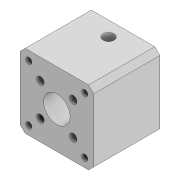
# Autodesk Inventor part: Part1_b
Saved by Autodesk Inventor 2021 (Build 250183000, 183)
## iProperties
Created: 2022-05-23
Part Number: Part1_b
Material: Generic
Document SubType Name: Modeling
Designer: romanp
Density: 1 g/cm^3
Appearance: Default
Author: romanp
Autodesk Inventor part; units mm, degrees
ref_plane "YZ Plane" through (0, 0, 0) normal (1, 0, 0) x (0, 1, 0)
ref_plane "XZ Plane" through (0, 0, 0) normal (0, 1, 0) x (-1, 0, 0)
ref_plane "XY Plane" through (0, 0, 0) normal (0, 0, 1) x (1, 0, 0)
sketch "Sketch11" plane through (0, 0, 0) normal (0, 0, 1) x (1, 0, 0)
  line L0 (-3.4593, 3.4593) -> (0, 0)
  line L1 (-3.4593, 3.4593) -> (-3.4593, 46.5407)
  line L2 (0, 50) -> (-3.4593, 46.5407)
  line L3 (43.0814, 50) -> (0, 50)
  line L4 (46.5407, 46.5407) -> (43.0814, 50)
  line L5 (46.5407, 3.4593) -> (46.5407, 46.5407)
  line L6 (43.0814, 0) -> (46.5407, 3.4593)
  line L7 (43.0814, 0) -> (0, 0)
  constraints: 16 end point
extrude "Extrusion8" add sketch "Sketch11" along normal blind 5
sketch "Sketch16" plane through (0, 0, 0) normal (0, 0, -1) x (-1, 0, 0)
  line L0 (-27.0407, 40) -> (-34.0407, 40)
  line L1 (-36.5407, 37.5) -> (-36.5407, 30.5)
  arc A0 (-34.0407, 40) -> (-36.5407, 37.5) centre (-34.0407, 37.5) ccw
  line L2 (-9.0407, 40) -> (-16.0407, 40)
  arc A1 (-6.5407, 37.5) -> (-9.0407, 40) centre (-9.0407, 37.5) ccw
  line L3 (-6.5407, 30.5) -> (-6.5407, 37.5)
  line L4 (-6.5407, 12.5) -> (-6.5407, 19.5)
  arc A2 (-9.0407, 10) -> (-6.5407, 12.5) centre (-9.0407, 12.5) ccw
  line L5 (-16.0407, 10) -> (-9.0407, 10)
  line L6 (-34.0407, 10) -> (-27.0407, 10)
  arc A3 (-36.5407, 12.5) -> (-34.0407, 10) centre (-34.0407, 12.5) ccw
  line L7 (-36.5407, 19.5) -> (-36.5407, 12.5)
  line L8 (0, 50) -> (3.4593, 46.5407) projected
  line L9 (-43.0814, 0) -> (-46.5407, 3.4593) projected
  line L10 (-46.5407, 46.5407) -> (-43.0814, 50) projected
  line L11 (-43.0814, 0) -> (-43.0814, 50)
  line L12 (3.4593, 3.4593) -> (0, 0) projected
  line L13 (-6.5407, 30.5) -> (-6.5407, 19.5)
  line L14 (-16.0407, 40) -> (-27.0407, 40)
  line L15 (-36.5407, 30.5) -> (-36.5407, 19.5)
  line L16 (-27.0407, 10) -> (-16.0407, 10)
  circle A4 centre (-2.5407, 44) radius 2.5
  circle A5 centre (-40.5407, 6) radius 2.5
  circle A6 centre (-2.5407, 6) radius 2.5
  circle A7 centre (-40.5407, 44) radius 2.5
  line L17 (0, 50) -> (3.4593, 46.5407)
  line L18 (3.4593, 46.5407) -> (3.4593, 3.4593) projected
  line L19 (0, 0) -> (-43.0814, 0) projected
  line L20 (3.4593, 3.4593) -> (0, 0)
  line L21 (0, 0) -> (-43.0814, 0)
  line L22 (-43.0814, 0) -> (-46.5407, 3.4593) projected
  line L23 (-43.0814, 0) -> (-46.5407, 3.4593)
  line L24 (-46.5407, 3.4593) -> (-46.5407, 46.5407) projected
  line L25 (-46.5407, 3.4593) -> (-46.5407, 46.5407)
  line L26 (-46.5407, 46.5407) -> (-43.0814, 50)
  line L27 (0, 50) -> (-43.0814, 50) projected
  line L28 (0, 50) -> (-43.0814, 50)
  dimension "d44" = 5
  dimension "d45" = 5
  dimension "d46" = 5
  dimension "d47" = 5
  constraints: 40 end point, 8 centre point, 8 collinear, 8 point on circle, 2 vertical, 1 perpendicular, 1 point on line
  measures "d44" diameter of A4
  measures "d45" diameter of A5
  measures "d46" diameter of A6
  measures "d47" diameter of A7
extrude "Extrusion11" add sketch "Sketch16" along normal blind 15
sketch "Sketch18" plane through (0, 0, -15) normal (0, 0, -1) x (-1, 0, 0)
  circle A0 centre (-2.5407, 6) radius 2.5 projected
  circle A1 centre (-2.5407, 6) radius 2.5
  circle A2 centre (-40.5407, 6) radius 2.5 projected
  circle A3 centre (-40.5407, 6) radius 2.5
  circle A4 centre (-40.5407, 44) radius 2.5 projected
  circle A5 centre (-40.5407, 44) radius 2.5
  circle A6 centre (-2.5407, 44) radius 2.5 projected
  circle A7 centre (-2.5407, 44) radius 2.5
  point P0 (0, 0)
  constraints: 4 centre point, 4 coincident
extrude "Extrusion12" cut sketch "Sketch18" against normal blind 100
sketch "Sketch19" plane through (0, 0, -15) normal (0, 0, -1) x (-1, 0, 0)
  circle A0 centre (-2.5407, 6) radius 2.5 projected
  circle A1 centre (-2.5407, 6) radius 4.3
  circle A2 centre (-40.5407, 6) radius 2.5 projected
  circle A3 centre (-40.5407, 6) radius 4.3
  circle A4 centre (-2.5407, 44) radius 2.5 projected
  circle A5 centre (-2.5407, 44) radius 4.3
  circle A6 centre (-40.5407, 44) radius 2.5 projected
  circle A7 centre (-40.5407, 44) radius 4.3
  point P0 (0, 0)
  dimension "d54" = 8.6
  dimension "d55" = 8.6
  dimension "d56" = 8.6
  dimension "d57" = 8.6
  constraints: 4 centre point, 4 coincident
  measures "d54" diameter of A1
  measures "d55" diameter of A3
  measures "d56" diameter of A5
  measures "d57" diameter of A7
extrude "Extrusion13" cut sketch "Sketch19" against normal blind 10 contours A0 | A1 | A2 | A3 | A5 | A6 | A7
sketch "Sketch20" plane through (0, 0, -15) normal (0, 0, -1) x (-1, 0, 0)
  line L0 (0, 50) -> (-43.0814, 50) projected
  line L1 (-43.0814, 50) -> (-46.5407, 46.5407) projected
  line L2 (-46.5407, 46.5407) -> (-46.5407, 3.4593) projected
  line L3 (-46.5407, 3.4593) -> (-43.0814, 0) projected
  line L4 (-43.0814, 0) -> (0, 0) projected
  line L5 (0, 0) -> (3.4593, 3.4593) projected
  line L6 (3.4593, 3.4593) -> (3.4593, 46.5407) projected
  line L7 (3.4593, 46.5407) -> (0, 50) projected
  circle A0 centre (-2.5407, 44) radius 4.3 projected
  circle A1 centre (-40.5407, 44) radius 4.3 projected
  circle A2 centre (-40.5407, 6) radius 4.3 projected
  circle A3 centre (-2.5407, 6) radius 4.3 projected
  arc A4 (-9.0407, 10) -> (-6.5407, 12.5) centre (-9.0407, 12.5) ccw projected
  line L8 (-9.0407, 10) -> (-34.0407, 10) projected
  line L9 (-36.5407, 12.5) -> (-36.5407, 37.5) projected
  arc A5 (-36.5407, 12.5) -> (-34.0407, 10) centre (-34.0407, 12.5) ccw projected
  line L10 (-6.5407, 37.5) -> (-6.5407, 12.5) projected
  arc A6 (-6.5407, 37.5) -> (-9.0407, 40) centre (-9.0407, 37.5) ccw projected
  line L11 (-34.0407, 40) -> (-9.0407, 40) projected
  arc A7 (-34.0407, 40) -> (-36.5407, 37.5) centre (-34.0407, 37.5) ccw projected
extrude "Extrusion14" add sketch "Sketch20" along normal blind 25
sketch "Sketch21" plane through (0, 50, 5) normal (0, 1, 0) x (1, 0, 0)
  line L0 (-1.7593, 45) -> (6.8407, 45) projected
  circle A0 centre (21.6907, 35) radius 2
  dimension "d63" = 4
  constraints: 1 centre point
  measures "d63" diameter of A0
extrude "Extrusion15" cut sketch "Sketch21" against normal blind 500
sketch "Sketch22" plane through (0, 50, 5) normal (0, 1, 0) x (1, 0, 0)
  circle A0 centre (21.6907, 35) radius 2 projected
  circle A1 centre (21.6907, 35) radius 3.75
  point P0 (0, 5)
  dimension "d67" = 7.5
  constraints: 1 centre point, 1 coincident
  measures "d67" diameter of A1
extrude "Extrusion16" cut sketch "Sketch22" against normal blind 5 contours A0 | A1
sketch "Sketch23" plane through (0, 0, 5) normal (0, -1, 0) x (1, 0, 0)
  circle A0 centre (21.6907, -35) radius 2 projected
  circle A1 centre (21.6907, -35) radius 3.75
  point P0 (0, -5)
  dimension "d70" = 7.5
  constraints: 1 centre point, 1 coincident
  measures "d70" diameter of A1
extrude "Extrusion17" cut sketch "Sketch23" against normal blind 5
sketch "Sketch25" plane through (2.5407, 44, -5) normal (0, 0, -1) x (-1, 0, 0)
  circle A0 centre (0, 0) radius 2.5 projected
  circle A1 centre (0, -38) radius 2.5 projected
  circle A2 centre (-38, -38) radius 2.5 projected
  circle A3 centre (-38, 0) radius 2.5 projected
  circle A4 centre (0, 0) radius 2
  circle A5 centre (0, -38) radius 2.5 projected
  circle A6 centre (0, -38) radius 2
  circle A7 centre (-38, -38) radius 2
  circle A8 centre (-38, 0) radius 2
  point P0 (2.5407, -44)
  dimension "d75" = 4
  dimension "d76" = 4
  dimension "d77" = 4
  dimension "d78" = 4
  constraints: 4 centre point, 4 coincident
  measures "d75" diameter of A4
  measures "d76" diameter of A6
  measures "d77" diameter of A7
  measures "d78" diameter of A8
extrude "Extrusion18" add sketch "Sketch25" against normal blind 10
sketch "Sketch26" plane through (0, 0, -40) normal (0, 0, -1) x (-1, 0, 0)
  circle A0 centre (-2.5407, 44) radius 4.3 projected
  circle A1 centre (-2.5407, 6) radius 4.3 projected
  circle A2 centre (-40.5407, 6) radius 4.3 projected
  circle A3 centre (-40.5407, 44) radius 4.3 projected
  circle A4 centre (-2.5407, 6) radius 2 projected
  circle A5 centre (-2.5407, 6) radius 3.8
  circle A6 centre (-40.5407, 6) radius 4.3 projected
  circle A7 centre (-40.5407, 6) radius 3.8
  circle A8 centre (-2.5407, 44) radius 2 projected
  circle A9 centre (-2.5407, 44) radius 3.8
  circle A10 centre (-40.5407, 44) radius 2 projected
  circle A11 centre (-40.5407, 44) radius 3.8
  point P0 (0, 0)
  dimension "d81" = 7.6
  dimension "d82" = 7.6
  dimension "d83" = 7.6
  dimension "d84" = 7.6
  constraints: 4 centre point, 4 coincident
  measures "d81" diameter of A5
  measures "d82" diameter of A7
  measures "d83" diameter of A9
  measures "d84" diameter of A11
extrude "Extrusion19" add sketch "Sketch26" against normal blind 35 contours A0 | A1 | A2 | A3
sketch "Sketch27" plane through (0, 0, 5) normal (0, 0, 1) x (1, 0, 0)
  circle A0 centre (2.5407, 44) radius 2 projected
  circle A1 centre (40.5407, 44) radius 2 projected
  circle A2 centre (2.5407, 6) radius 2 projected
  circle A3 centre (40.5407, 6) radius 2 projected
  circle A4 centre (21.5407, 25) radius 9
  point P0 (0, 0)
  dimension "d88" = 18
  constraints: 1 centre point
  measures "d88" diameter of A4
extrude "Extrusion20" cut sketch "Sketch27" against normal blind 35 contours A4
sketch "Sketch32" plane through (0, 0, -40) normal (0, 0, -1) x (-1, 0, 0)
  circle A0 centre (-21.5407, 25) radius 9 projected
  circle A1 centre (-2.5407, 6) radius 2 projected
  circle A2 centre (-40.5407, 44) radius 2 projected
  circle A3 centre (-2.5407, 44) radius 2 projected
  circle A4 centre (-40.5407, 6) radius 2 projected
  circle A5 centre (-10.4038, 13.8631) radius 2.5
  circle A6 centre (-32.6776, 13.8631) radius 2.5
  circle A7 centre (-10.4038, 36.1369) radius 2.5
  circle A8 centre (-32.6776, 36.1369) radius 2.5
  point P0 (0, 0)
  dimension "d93" = 5
  dimension "d94" = 5
  dimension "d95" = 5
  dimension "d96" = 5
  constraints: 4 centre point
  measures "d93" diameter of A5
  measures "d94" diameter of A6
  measures "d95" diameter of A7
  measures "d96" diameter of A8
extrude "Extrusion21" cut sketch "Sketch32" against normal blind 100 contours A5 | A6 | A7 | A8
sketch "Sketch33" plane through (0, 0, 0) normal (0, 0, -1) x (-1, 0, 0)
  circle A0 centre (-10.4038, 13.8631) radius 2.5 projected
  circle A1 centre (-10.4038, 13.8631) radius 4.5
  circle A2 centre (-10.4038, 36.1369) radius 2.5 projected
  circle A3 centre (-10.4038, 36.1369) radius 4.5
  circle A4 centre (-32.6776, 36.1369) radius 2.5 projected
  circle A5 centre (-32.6776, 36.1369) radius 4.5
  circle A6 centre (-32.6776, 13.8631) radius 2.5 projected
  circle A7 centre (-32.6776, 13.8631) radius 4.5
  point P0 (0, 0)
  dimension "d99" = 9
  dimension "d100" = 9
  dimension "d101" = 9
  dimension "d102" = 9
  constraints: 4 centre point, 4 coincident
  measures "d99" diameter of A1
  measures "d100" diameter of A3
  measures "d101" diameter of A5
  measures "d102" diameter of A7
extrude "Extrusion22" cut sketch "Sketch33" along normal blind 100 and the other way blind 5
sketch "Sketch34" plane through (0, 0, 5) normal (0, 0, 1) x (1, 0, 0)
  circle A0 centre (10.4038, 36.1369) radius 4.5 projected
  circle A1 centre (10.4038, 36.1369) radius 2.5
  arc A2 (30.3697, 40) -> (36.5407, 33.829) centre (32.6776, 36.1369) ccw projected
  circle A3 centre (32.6776, 36.1369) radius 2.5
  circle A4 centre (10.4038, 13.8631) radius 4.5 projected
  circle A5 centre (10.4038, 13.8631) radius 2.5
  circle A6 centre (32.6776, 13.8631) radius 4.5 projected
  circle A7 centre (32.6776, 13.8631) radius 2.5
  circle A8 centre (32.6776, 36.1369) radius 4.5 projected
  point P0 (0, 0)
  dimension "d107" = 5
  dimension "d108" = 5
  dimension "d109" = 5
  dimension "d110" = 5
  constraints: 4 centre point, 4 coincident
  measures "d107" diameter of A1
  measures "d108" diameter of A3
  measures "d109" diameter of A5
  measures "d110" diameter of A7
extrude "Extrusion23" add sketch "Sketch34" against normal blind 5
sketch "Sketch35" plane through (0, 0, 0) normal (0, 0, -1) x (-1, 0, 0)
  circle A0 centre (-32.6776, 13.8631) radius 2.5 projected
  circle A1 centre (-32.6776, 36.1369) radius 2.5 projected
  circle A2 centre (-10.4038, 13.8631) radius 2.5 projected
  circle A3 centre (-10.4038, 36.1369) radius 2.5 projected
  line L0 (-30.3697, 10) -> (-12.7117, 10) projected
  arc A4 (-12.7117, 10) -> (-6.5407, 16.171) centre (-10.4038, 13.8631) ccw projected
  line L1 (-6.5407, 16.171) -> (-6.5407, 33.829) projected
  arc A5 (-6.5407, 33.829) -> (-12.7117, 40) centre (-10.4038, 36.1369) ccw projected
  line L2 (-12.7117, 40) -> (-30.3697, 40) projected
  arc A6 (-30.3697, 40) -> (-36.5407, 33.829) centre (-32.6776, 36.1369) ccw projected
  line L3 (-36.5407, 33.829) -> (-36.5407, 16.171) projected
  arc A7 (-36.5407, 16.171) -> (-30.3697, 10) centre (-32.6776, 13.8631) ccw projected
  circle A8 centre (-21.5407, 25) radius 9 projected
  circle A9 centre (-32.6776, 36.1369) radius 4.5
  circle A10 centre (-10.4038, 36.1369) radius 2.5 projected
  circle A11 centre (-10.4038, 36.1369) radius 4.5
  circle A12 centre (-32.6776, 13.8631) radius 4.5
  circle A13 centre (-10.4038, 13.8631) radius 2.5 projected
  arc A14 (-12.7117, 10) -> (-6.5407, 16.171) centre (-10.4038, 13.8631) ccw projected
  circle A15 centre (-10.4038, 13.8631) radius 4.5
  point P0 (0, 0)
  point P1 (-12.7117, 40)
  constraints: 4 coincident, 2 centre point, 6 other
extrude "Extrusion24" add sketch "Sketch35" along normal blind 10 contours A12 L3 A9 L2 A11 L1 A15 L0
sketch "Sketch37" plane through (40.5407, 44, -5) normal (0, 0, -1) x (-1, 0, 0)
  circle A0 centre (0, 0) radius 3.8 projected
  circle A1 centre (0, 0) radius 2 projected
  circle A2 centre (38, 0) radius 3.8 projected
  circle A3 centre (38, 0) radius 2 projected
  circle A4 centre (38, -38) radius 3.8 projected
  circle A5 centre (38, -38) radius 2 projected
  circle A6 centre (0, -38) radius 3.8 projected
  circle A7 centre (0, -38) radius 2 projected
  point P0 (40.5407, -44)
extrude "Extrusion25" add sketch "Sketch37" along normal blind 2
sketch "Sketch38" plane through (0, 0, -40) normal (0, 0, -1) x (-1, 0, 0)
  line L0 (-6.5407, 33.829) -> (-6.5407, 16.171) projected
  arc A0 (-12.7117, 40) -> (-6.5407, 33.829) centre (-10.4038, 36.1369) ccw projected
  line L1 (-30.3697, 40) -> (-12.7117, 40) projected
  arc A1 (-36.5407, 33.829) -> (-30.3697, 40) centre (-32.6776, 36.1369) ccw projected
  line L2 (-36.5407, 16.171) -> (-36.5407, 33.829) projected
  arc A2 (-30.3697, 10) -> (-36.5407, 16.171) centre (-32.6776, 13.8631) ccw projected
  line L3 (-12.7117, 10) -> (-30.3697, 10) projected
  arc A3 (-6.5407, 16.171) -> (-12.7117, 10) centre (-10.4038, 13.8631) ccw projected
  circle A4 centre (-21.5407, 25) radius 9 projected
  arc A5 (-30.3697, 40) -> (-36.5407, 33.829) centre (-32.6776, 36.1369) ccw projected
  arc A6 (-36.5407, 16.171) -> (-30.3697, 10) centre (-32.6776, 13.8631) ccw projected
  arc A7 (-6.5407, 33.829) -> (-12.7117, 40) centre (-10.4038, 36.1369) ccw projected
  line L4 (-36.5407, 16.171) -> (-36.5407, 33.829) projected
  arc A8 (-12.7117, 10) -> (-6.5407, 16.171) centre (-10.4038, 13.8631) ccw projected
  line L5 (-21.5407, 25) -> (-36.7907, 25)
  line L6 (-36.7907, 25) -> (-36.7907, 9.75)
  line L7 (-21.5407, 25) -> (-6.2907, 25)
  line L8 (-6.2907, 25) -> (-6.2907, 40.25)
  line L9 (-36.7907, 9.75) -> (-6.2907, 9.75)
  line L10 (-6.2907, 9.75) -> (-6.2907, 40.25)
  line L11 (-6.2907, 40.25) -> (-36.7907, 40.25)
  line L12 (-36.7907, 40.25) -> (-36.7907, 9.75)
  point P0 (0, 0)
  point P1 (-6.2907, 15.6886)
  point P2 (-6.2907, 34.3114)
  point P3 (-30.8521, 9.75)
  point P4 (-12.2293, 9.75)
  point P5 (-36.7907, 34.3114)
  point P6 (-36.7907, 15.6886)
  point P7 (-12.2293, 40.25)
  point P8 (-30.8521, 40.25)
  dimension "d122" = 15.25
  dimension "d123" = 15.25
  dimension "d124" = 15.25
  dimension "d125" = 15.25
  constraints: 16 end point, 3 horizontal, 2 parallel, 2 perpendicular, 1 vertical
  measures "d122" distance of L5.start L5.end
  measures "d123" distance of L5.end L6.end
  measures "d124" distance of L5.start L7.end
  measures "d125" distance of L7.end L8.end
extrude "Extrusion26" cut sketch "Sketch38" against normal blind 30 contours A7 L8 L7 L0 | L7 L10 A8 L0 | L1 A5 L11 A7 | A8 L9 A6 L3 | L2 L5 L12 A5 | L2 A6 L6 L5
sketch "Sketch41" plane through (21.6907, 5, -30) normal (0, -1, 0) x (1, 0, 0)
  circle A0 centre (0, 0) radius 2.05
  point P0 (-21.6907, 30)
  dimension "d130" = 4.1
  constraints: 1 centre point
  measures "d130" diameter of A0
extrude "Extrusion28" cut sketch "Sketch41" against normal blind 100
sketch "Sketch42" plane through (0, 0, -40) normal (0, 0, -1) x (-1, 0, 0)
  circle A0 centre (-40.5407, 44) radius 2 projected
  circle A1 centre (-40.5407, 44) radius 2.05
  circle A2 centre (-2.5407, 44) radius 2 projected
  circle A3 centre (-2.5407, 44) radius 2.05
  circle A4 centre (-40.5407, 6) radius 2 projected
  circle A5 centre (-40.5407, 6) radius 2.05
  circle A6 centre (-2.5407, 6) radius 2 projected
  circle A7 centre (-2.5407, 6) radius 2.05
  circle A8 centre (-10.4038, 36.1369) radius 2.5 projected
  circle A9 centre (-10.4038, 36.1369) radius 2.55
  circle A10 centre (-32.6776, 36.1369) radius 2.5 projected
  circle A11 centre (-32.6776, 36.1369) radius 2.55
  circle A12 centre (-32.6776, 13.8631) radius 2.5 projected
  circle A13 centre (-32.6776, 13.8631) radius 2.55
  circle A14 centre (-10.4038, 13.8631) radius 2.5 projected
  circle A15 centre (-10.4038, 13.8631) radius 2.55
  point P0 (0, 0)
  dimension "d133" = 4.1
  dimension "d134" = 4.1
  dimension "d135" = 4.1
  dimension "d136" = 4.1
  dimension "d137" = 5.1
  dimension "d138" = 5.1
  dimension "d139" = 5.1
  dimension "d140" = 5.1
  constraints: 8 centre point, 8 coincident
  measures "d133" diameter of A1
  measures "d134" diameter of A3
  measures "d135" diameter of A5
  measures "d136" diameter of A7
  measures "d137" diameter of A9
  measures "d138" diameter of A11
  measures "d139" diameter of A13
  measures "d140" diameter of A15
extrude "Extrusion29" cut sketch "Sketch42" against normal blind 100 contours A0 | A1 | A2 | A3 | A4 | A5 | A6 | A7 | A8 | A9 | A10 | A11 | A12 | A13 | A14 | A15
sketch "Sketch43" plane through (0, 0, -40) normal (0, 0, -1) x (-1, 0, 0)
  arc A0 (-34.2919, 40.3015) -> (-36.8422, 37.7513) centre (-34.2919, 37.7513) ccw
  line L0 (-36.8422, 12.2488) -> (-36.8422, 37.7513)
  line L1 (-34.2919, 40.3015) -> (-8.7894, 40.3015)
  arc A1 (-36.8422, 12.2488) -> (-34.292, 9.6985) centre (-34.292, 12.2488) ccw
  line L2 (-8.7895, 9.6985) -> (-34.292, 9.6985)
  line L3 (-6.2392, 37.7512) -> (-6.2392, 12.2487)
  arc A2 (-8.7895, 9.6985) -> (-6.2392, 12.2487) centre (-8.7895, 12.2487) ccw
  arc A3 (-6.2392, 37.7512) -> (-8.7894, 40.3015) centre (-8.7895, 37.7512) ccw
  circle A4 centre (-21.5407, 25) radius 9
  circle A5 centre (-21.5407, 25) radius 1
  point P0 (0, 0)
  dimension "d143" = 2
  constraints: 8 end point, 8 point on circle, 6 centre point
  measures "d143" diameter of A5
extrude "Extrusion30" cut sketch "Sketch43" against normal blind 30 contours L1 A3 L3 A2 L2 A1 L0 A0 | A4 | A5
sketch "Sketch44" plane through (0, 0, -40) normal (0, 0, -1) x (-1, 0, 0)
  arc A0 (-6.241, 37.846) -> (-8.6947, 40.2997) centre (-10.4038, 36.1369) ccw projected
  arc A1 (-6.241, 37.846) -> (-8.6947, 40.2997) centre (-8.7895, 37.7512) ccw projected
  arc A2 (-34.3867, 40.2997) -> (-36.8404, 37.846) centre (-32.6776, 36.1369) ccw projected
  arc A3 (-34.3867, 40.2997) -> (-36.8404, 37.846) centre (-34.2919, 37.7513) ccw projected
  arc A4 (-36.8404, 12.154) -> (-34.3867, 9.7003) centre (-32.6776, 13.8631) ccw projected
  arc A5 (-36.8404, 12.154) -> (-34.3867, 9.7003) centre (-34.292, 12.2488) ccw projected
  arc A6 (-8.6947, 9.7003) -> (-6.241, 12.154) centre (-10.4038, 13.8631) ccw projected
  arc A7 (-8.6947, 9.7003) -> (-6.241, 12.154) centre (-8.7895, 12.2487) ccw projected
  point P0 (0, 0)
extrude "Extrusion31" cut sketch "Sketch44" against normal blind 40
body "Solid2"
